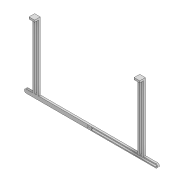
# Autodesk Inventor part: Bancada
Saved by Autodesk Inventor 2021 (Build 250183000, 183)
## iProperties
Created: 2021-04-19
Part Number: Bancada
Material: Genérico
Document SubType Name: Modeling
Designer: carlo
Density: 1 g/cm^3
Appearance: Valor por defecto
Mass: 32.5704 g
Surface Area: 255.981 cm^2
Volume: 32.5704 cm^3
Author: carlo
Autodesk Inventor part; units mm, degrees
ref_plane "YZ Plane" through (0, 0, 0) normal (1, 0, 0) x (0, 1, 0)
ref_plane "XZ Plane" through (0, 0, 0) normal (0, 1, 0) x (-1, 0, 0)
ref_plane "XY Plane" through (0, 0, 0) normal (0, 0, 1) x (1, 0, 0)
sketch "Boceto1" plane through (0, 0, 0) normal (0, 0, 1) x (1, 0, 0)
  line L0 (5, -5) -> (165, -5)
  line L1 (165, -2.5) -> (8, -2.5)
  line L2 (8, -2.5) -> (8, 2.5)
  line L3 (8, 2.5) -> (165, 2.5)
  line L4 (140, 5) -> (142.5, 5)
  line L5 (142.5, 5) -> (137.5, 5)
  line L6 (137.5, 5) -> (137.5, 180)
  line L7 (142.5, 180) -> (142.5, 5)
  line L8 (132.5, 185) -> (147.5, 185)
  line L9 (147.5, 185) -> (147.5, 5)
  line L10 (142.5, 5) -> (137.5, 5)
  line L11 (132.5, 5) -> (132.5, 185)
  line L12 (137.5, 180) -> (142.5, 180)
  line L13 (147.5, 5) -> (165, 5)
  line L14 (0, 5) -> (132.5, 5)
  line L15 (137.5, 5) -> (142.5, 5)
  arc A0 (-165, 5) -> (-165, -5) centre (-165, 0) ccw
  line L16 (5, -5) -> (-165, -5)
  line L17 (-140, 5) -> (-142.5, 5)
  line L18 (-142.5, 5) -> (-137.5, 5)
  line L19 (-137.5, 5) -> (-137.5, 180)
  line L20 (-142.5, 180) -> (-142.5, 5)
  line L21 (-132.5, 185) -> (-147.5, 185)
  line L22 (-147.5, 185) -> (-147.5, 5)
  line L23 (-142.5, 5) -> (-137.5, 5)
  line L24 (-132.5, 5) -> (-132.5, 185)
  line L25 (-137.5, 180) -> (-142.5, 180)
  line L26 (-147.5, 5) -> (-165, 5)
  line L27 (0, 5) -> (-132.5, 5)
  line L28 (-137.5, 5) -> (-142.5, 5)
  line L29 (0, 0) -> (-5, 0) construction
  circle A1 centre (0, 0) radius 2.5
  arc A2 (180, -2.5) -> (180, 2.5) centre (180, 0) ccw
  line L30 (180, 5) -> (165, 5)
  line L31 (165, 2.5) -> (180, 2.5)
  line L32 (165, -2.5) -> (180, -2.5)
  line L33 (165, -5) -> (180, -5)
  arc A3 (180, -5) -> (180, 5) centre (180, 0) ccw
  dimension "d13" = 15
  dimension "d17" = 180
  dimension "d18" = 175
  dimension "d31" = 10
  dimension "d36" = 5
  dimension "d40" = 5
  constraints: 68 end point, 8 parallel, 6 horizontal, 6 point on circle, 4 centre point, 4 perpendicular, 2 coincident, 2 tangent
  measures "d13" distance of L9.end L11.start
  measures "d17" distance of L11.start L8.start
  measures "d18" distance between parallel lines of L14 L12
  measures "d31" distance between parallel lines of L27 L16
  measures "d36" diameter of A1
  measures "d40" diameter of A2
extrude "Extrusión1" add sketch "Boceto1" along normal blind 5
sketch "Sketch4" plane through (0, 0, 5) normal (0, 0, 1) x (1, 0, 0)
  line L0 (-132.5, 185) -> (-147.5, 185) projected
  line L1 (-132.5, 5) -> (-132.5, 185) projected
  line L2 (-147.5, 185) -> (-132.5, 185)
  line L3 (-132.5, 185) -> (-132.5, 180)
  line L4 (-132.5, 180) -> (-147.5, 180)
  line L5 (-147.5, 180) -> (-147.5, 185)
  line L6 (180, 5) -> (147.5, 5) projected
  line L7 (147.5, 5) -> (147.5, 185) projected
  line L8 (147.5, 185) -> (132.5, 185) projected
  line L9 (132.5, 185) -> (132.5, 5) projected
  line L10 (132.5, 5) -> (-132.5, 5) projected
  line L11 (-132.5, 5) -> (-132.5, 185) projected
  line L12 (-132.5, 185) -> (-147.5, 185) projected
  line L13 (-147.5, 185) -> (-147.5, 5) projected
  line L14 (-147.5, 5) -> (-165, 5) projected
  arc A0 (-165, 5) -> (-165, -5) centre (-165, 0) ccw projected
  line L15 (-165, -5) -> (180, -5) projected
  line L16 (-142.5, 5) -> (-142.5, 180) projected
  line L17 (-142.5, 180) -> (-137.5, 180) projected
  line L18 (-137.5, 180) -> (-137.5, 5) projected
  line L19 (-137.5, 5) -> (-142.5, 5) projected
  line L20 (142.5, 180) -> (142.5, 5) projected
  line L21 (142.5, 5) -> (137.5, 5) projected
  line L22 (137.5, 5) -> (137.5, 180) projected
  line L23 (137.5, 180) -> (142.5, 180) projected
  line L24 (132.5, 185) -> (147.5, 185)
  line L25 (147.5, 185) -> (147.5, 180)
  line L26 (147.5, 180) -> (132.5, 180)
  line L27 (132.5, 180) -> (132.5, 185)
  arc A1 (180, -5) -> (180, 5) centre (180, 0) ccw projected
  point P0 (0, 0)
  dimension "d26" = 5
  constraints: 16 end point, 4 parallel, 2 horizontal, 2 perpendicular, 2 point on line
  measures "d26" distance of L2.end L3.end
extrude "Extrusion3" add sketch "Sketch4" along normal blind 10 contours L1 L4 L5 L0 | L9 L8 L7 L26 L23
